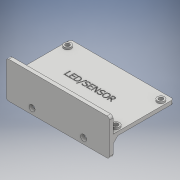
# Autodesk Inventor part: Eletronica - suporteLed
Saved by Autodesk Inventor 2017 (Build 210142000, 142)
## iProperties
Created: 2020-10-10
Part Number: Eletronica - suporteLed
Material: Generic
Document SubType Name: Modeling
Designer: ale
Density: 1 g/cm^3
Appearance: Default
Author: ale
Autodesk Inventor part; units mm, degrees
ref_plane "YZ Plane" through (0, 0, 0) normal (1, 0, 0) x (0, 1, 0)
ref_plane "XZ Plane" through (0, 0, 0) normal (0, 1, 0) x (-1, 0, 0)
ref_plane "XY Plane" through (0, 0, 0) normal (0, 0, 1) x (1, 0, 0)
sketch "Sketch1" plane through (0, 0, 0) normal (0, 0, 1) x (1, 0, 0)
  line L0 (-42.5, 25) -> (42.5, 25)
  line L1 (42.5, 25) -> (42.5, -25)
  line L2 (42.5, -25) -> (-42.5, -25)
  line L3 (-42.5, -25) -> (-42.5, 25)
  line L4 (-42.5, 25) -> (42.5, -25) construction
  line L5 (42.5, 25) -> (-42.5, -25) construction
  point P0 (0, 0)
  dimension "d0" = 85
  dimension "d1" = 50
  constraints: 12 end point, 2 midpoint, 2 parallel, 1 horizontal, 1 perpendicular
  measures "d0" distance of L1.end L2.end
  measures "d1" distance of L0.end L1.end
extrude "Extrusion1" add sketch "Sketch1" along normal blind 3
sketch "Sketch2" plane through (0, 0, 3) normal (0, 0, 1) x (1, 0, 0)
  line L0 (-38.5, 18.5) -> (38.5, 18.5)
  line L1 (38.5, 18.5) -> (38.5, -18.5)
  line L2 (38.5, -18.5) -> (-38.5, -18.5)
  line L3 (-38.5, -18.5) -> (-38.5, 18.5)
  line L4 (-38.5, 18.5) -> (38.5, -18.5) construction
  line L5 (38.5, 18.5) -> (-38.5, -18.5) construction
  circle A0 centre (-38.5, 18.5) radius 3
  circle A1 centre (38.5, 18.5) radius 3
  circle A2 centre (38.5, -18.5) radius 3
  circle A3 centre (-38.5, -18.5) radius 3
  point P0 (0, 0)
  dimension "d30" = 5
  dimension "d4" = 77
  dimension "d5" = 37
  dimension "d6" = 6
  dimension "d7" = 6
  dimension "d8" = 6
  dimension "d9" = 6
  constraints: 12 end point, 4 centre point, 4 coincident, 2 midpoint, 2 parallel, 1 horizontal, 1 perpendicular
  measures "d4" distance of L1.end L2.end
  measures "d5" distance of L0.end L1.end
  measures "d6" diameter of A0
  measures "d7" diameter of A1
  measures "d8" diameter of A2
  measures "d9" diameter of A3
extrude "Extrusion2" add sketch "Sketch2" along normal blind 1.5 contours L3 A0 L0 | L0 A0 L3 | A1 L1 L0 | L0 L1 A1 | A3 L2 L3 | L3 L2 A3 | A2 L2 L1 | L1 L2 A2
sketch "Sketch3" plane through (-38.5, 18.5, 4.5) normal (0, 0, 1) x (1, 0, 0)
  circle A0 centre (0, 0) radius 3 projected
  circle A1 centre (77, 0) radius 3 projected
  circle A2 centre (77, -37) radius 3 projected
  circle A3 centre (0, -37) radius 3 projected
  point P0 (38.5, -18.5)
  constraints: 4 coincident
hole "Hole1" at (-38.5, 18.5, 4.5) at (38.5, 18.5, 4.5) at (38.5, -18.5, 4.5) at (-38.5, -18.5, 4.5) direction (0, 0, -1) diameter 3.5 end through all
sketch "Sketch4" plane through (-42.5, -25, 0) normal (0, -1, 0) x (1, 0, 0)
  line L0 (0, 0) -> (0, 3) projected
  line L1 (0, 1.5) -> (85, 1.5)
  line L2 (85, 0) -> (0, 0) projected
  line L3 (0, 16.5) -> (85, 16.5)
  line L4 (85, 16.5) -> (85, -13.5)
  line L5 (85, -13.5) -> (0, -13.5)
  line L6 (0, -13.5) -> (0, 16.5)
  line L7 (0, 16.5) -> (85, -13.5) construction
  line L8 (85, 16.5) -> (0, -13.5) construction
  point P0 (42.5, 0)
  point P1 (42.5, 1.5)
  dimension "d19" = 85
  dimension "d20" = 30
  constraints: 14 end point, 4 midpoint, 3 parallel, 1 horizontal, 1 perpendicular
  measures "d19" distance of L4.end L5.end
  measures "d20" distance of L3.end L4.end
extrude "Extrusion3" add sketch "Sketch4" along normal blind 3
chamfer "Chamfer1" distance 4 angle 45 1 edges at (0, -25, 0)
sketch "Sketch5" plane through (-42.5, -25, 0) normal (0, 1, 0) x (1, 0, 0)
  line L0 (85, 13.5) -> (0, 13.5) projected
  line L1 (85, 4) -> (85, 13.5) projected
  point P0 (42.5, 0)
  point P1 (63.75, 8.75)
  point P2 (21.25, 8.75)
  dimension "d26" = 4.75
  dimension "d27" = 4.75
  dimension "d28" = 21.25
  dimension "d29" = 63.75
  measures "d26" distance from line of L0 point (63.75, 8.75)
  measures "d27" distance from line of L0 point (21.25, 8.75)
  measures "d28" distance from line of L1 point (63.75, 8.75)
  measures "d29" distance from line of point (21.25, 8.75) L1
hole "Hole2" at (21.25, -25, -8.75) at (-21.25, -25, -8.75) direction (0, -1, 0) diameter 5 end through all
fillet "Fillet1" radius 2 6 edges at (42.5, 25, 1.5) (-42.5, 25, 1.5) (-42.5, -26.5, -13.5) (42.5, -26.5, -13.5) (42.5, -26.5, 16.5) (-42.5, -26.5, 16.5)
sketch "Sketch6" plane through (0, 0, 3) normal (0, 0, 1) x (1, 0, 0)
  line L0 (-20.993, 2.6241) -> (18.8165, 2.6241) construction
  line L1 (18.8165, 2.6241) -> (18.8165, -3.6846) construction
  line L2 (18.8165, -3.6846) -> (-20.993, -3.6846) construction
  line L3 (-20.993, -3.6846) -> (-20.993, 2.6241) construction
  line L4 (-17.5895, -2.5987) -> (-20.4866, -2.5987)
  line L5 (-20.4866, -2.5987) -> (-20.4866, 2.4013)
  line L6 (-20.4866, 2.4013) -> (-19.8221, 2.4013)
  line L7 (-19.8221, 2.4013) -> (-19.8221, -2.0072)
  line L8 (-19.8221, -2.0072) -> (-17.5895, -2.0072)
  line L9 (-17.5895, -2.0072) -> (-17.5895, -2.5987)
  line L10 (-17.0668, -2.5987) -> (-17.0668, 2.4013)
  line L11 (-17.0668, 2.4013) -> (-13.9387, 2.4013)
  line L12 (-13.9387, 2.4013) -> (-13.9387, 1.8097)
  line L13 (-13.9387, 1.8097) -> (-16.4023, 1.8097)
  line L14 (-16.4023, 1.8097) -> (-16.4023, 0.4402)
  line L15 (-16.4023, 0.4402) -> (-14.1049, 0.4402)
  line L16 (-14.1049, 0.4402) -> (-14.1049, -0.1514)
  line L17 (-14.1049, -0.1514) -> (-16.4023, -0.1514)
  line L18 (-16.4023, -0.1514) -> (-16.4023, -2.0072)
  line L19 (-16.4023, -2.0072) -> (-13.9387, -2.0072)
  line L20 (-13.9387, -2.0072) -> (-13.9387, -2.5987)
  line L21 (-13.9387, -2.5987) -> (-17.0668, -2.5987)
  spline S0 degree 2 poles (-9.2669, -0.1028) (-9.2669, -0.7875) (-9.8221, -1.8896) (-10.288, -2.1976) knots 0 0 0 1 2 2 2
  spline S1 degree 2 poles (-10.288, -2.1976) (-10.6689, -2.4366) (-11.4509, -2.5987) (-12.0587, -2.5987) knots 0 0 0 1 2 2 2
  line L22 (-12.0587, -2.5987) -> (-13.2094, -2.5987)
  line L23 (-13.2094, -2.5987) -> (-13.2094, 2.4013)
  line L24 (-13.2094, 2.4013) -> (-12.0708, 2.4013)
  spline S2 degree 2 poles (-12.0708, 2.4013) (-11.3658, 2.4013) (-10.5635, 2.1906) (-10.2799, 2.0042) knots 0 0 0 1 2 2 2
  spline S3 degree 2 poles (-10.2799, 2.0042) (-9.7977, 1.6841) (-9.2669, 0.6266) (-9.2669, -0.1028) knots 0 0 0 1 2 2 2
  spline S4 degree 2 poles (-9.9598, -0.0947) (-9.9598, 0.4807) (-10.3407, 1.2951) (-10.7175, 1.5261) knots 0 0 0 1 2 2 2
  spline S5 degree 2 poles (-10.7175, 1.5261) (-10.9849, 1.6841) (-11.5887, 1.8259) (-12.0384, 1.8259) knots 0 0 0 1 2 2 2
  line L25 (-12.0384, 1.8259) -> (-12.5449, 1.8259)
  line L26 (-12.5449, 1.8259) -> (-12.5449, -2.0234)
  line L27 (-12.5449, -2.0234) -> (-12.0384, -2.0234)
  spline S6 degree 2 poles (-12.0384, -2.0234) (-11.5968, -2.0234) (-10.9282, -1.8815) (-10.6567, -1.6911) knots 0 0 0 1 2 2 2
  spline S7 degree 2 poles (-10.6567, -1.6911) (-10.3083, -1.4561) (-9.9598, -0.6781) (-9.9598, -0.0947) knots 0 0 0 1 2 2 2
  line L28 (-6.6089, 2.6241) -> (-8.566, -3.6846)
  line L29 (-8.566, -3.6846) -> (-9.1332, -3.6846)
  line L30 (-9.1332, -3.6846) -> (-7.1843, 2.6241)
  line L31 (-7.1843, 2.6241) -> (-6.6089, 2.6241)
  spline S8 degree 2 poles (-4.5222, -2.6879) (-5.0652, -2.6879) (-5.8269, -2.461) (-6.1632, -2.2989) knots 0 0 0 1 2 2 2
  line L32 (-6.1632, -2.2989) -> (-6.1632, -1.4642)
  line L33 (-6.1632, -1.4642) -> (-6.1146, -1.4642)
  spline S9 degree 2 poles (-6.1146, -1.4642) (-5.7864, -1.7721) (-4.9558, -2.1125) (-4.5708, -2.1125) knots 0 0 0 1 2 2 2
  spline S10 degree 2 poles (-4.5708, -2.1125) (-4.0198, -2.1125) (-3.4566, -1.6546) (-3.4566, -1.2778) knots 0 0 0 1 2 2 2
  spline S11 degree 2 poles (-3.4566, -1.2778) (-3.4566, -0.978) (-3.7524, -0.6052) (-4.0725, -0.512) knots 0 0 0 1 2 2 2
  spline S12 degree 2 poles (-4.0725, -0.512) (-4.3034, -0.4472) (-4.6883, -0.358) (-4.976, -0.2851) knots 0 0 0 1 2 2 2
  spline S13 degree 2 poles (-4.976, -0.2851) (-5.2353, -0.2162) (-5.6446, -0.0096) (-5.8026, 0.1565) knots 0 0 0 1 2 2 2
  spline S14 degree 2 poles (-5.8026, 0.1565) (-5.9566, 0.3227) (-6.1268, 0.7684) (-6.1268, 1.0601) knots 0 0 0 1 2 2 2
  spline S15 degree 2 poles (-6.1268, 1.0601) (-6.1268, 1.6679) (-5.1786, 2.4904) (-4.4452, 2.4904) knots 0 0 0 1 2 2 2
  spline S16 degree 2 poles (-4.4452, 2.4904) (-4.0238, 2.4904) (-3.2783, 2.3243) (-2.9582, 2.1663) knots 0 0 0 1 2 2 2
  line L34 (-2.9582, 2.1663) -> (-2.9582, 1.3721)
  line L35 (-2.9582, 1.3721) -> (-3.0068, 1.3721)
  spline S17 degree 2 poles (-3.0068, 1.3721) (-3.2459, 1.5909) (-3.9914, 1.9151) (-4.4007, 1.9151) knots 0 0 0 1 2 2 2
  spline S18 degree 2 poles (-4.4007, 1.9151) (-4.8626, 1.9151) (-5.4339, 1.4815) (-5.4339, 1.129) knots 0 0 0 1 2 2 2
  spline S19 degree 2 poles (-5.4339, 1.129) (-5.4339, 0.8129) (-5.0976, 0.4361) (-4.7815, 0.351) knots 0 0 0 1 2 2 2
  spline S20 degree 2 poles (-4.7815, 0.351) (-4.5708, 0.2943) (-3.959, 0.1484) (-3.7564, 0.0877) knots 0 0 0 1 2 2 2
  spline S21 degree 2 poles (-3.7564, 0.0877) (-3.2418, -0.0704) (-2.7637, -0.7065) (-2.7637, -1.1725) knots 0 0 0 1 2 2 2
  spline S22 degree 2 poles (-2.7637, -1.1725) (-2.7637, -1.4683) (-3.0028, -2.0355) (-3.2175, -2.2341) knots 0 0 0 1 2 2 2
  spline S23 degree 2 poles (-3.2175, -2.2341) (-3.4566, -2.4529) (-4.0644, -2.6879) (-4.5222, -2.6879) knots 0 0 0 1 2 2 2
  line L36 (-2.087, -2.5987) -> (-2.087, 2.4013)
  line L37 (-2.087, 2.4013) -> (1.041, 2.4013)
  line L38 (1.041, 2.4013) -> (1.041, 1.8097)
  line L39 (1.041, 1.8097) -> (-1.4225, 1.8097)
  line L40 (-1.4225, 1.8097) -> (-1.4225, 0.4402)
  line L41 (-1.4225, 0.4402) -> (0.8749, 0.4402)
  line L42 (0.8749, 0.4402) -> (0.8749, -0.1514)
  line L43 (0.8749, -0.1514) -> (-1.4225, -0.1514)
  line L44 (-1.4225, -0.1514) -> (-1.4225, -2.0072)
  line L45 (-1.4225, -2.0072) -> (1.041, -2.0072)
  line L46 (1.041, -2.0072) -> (1.041, -2.5987)
  line L47 (1.041, -2.5987) -> (-2.087, -2.5987)
  line L48 (5.3481, -2.5987) -> (4.6026, -2.5987)
  line L49 (4.6026, -2.5987) -> (2.3903, 1.7125)
  line L50 (2.3903, 1.7125) -> (2.3903, -2.5987)
  line L51 (2.3903, -2.5987) -> (1.7703, -2.5987)
  line L52 (1.7703, -2.5987) -> (1.7703, 2.4013)
  line L53 (1.7703, 2.4013) -> (2.7144, 2.4013)
  line L54 (2.7144, 2.4013) -> (4.7282, -1.5574)
  line L55 (4.7282, -1.5574) -> (4.7282, 2.4013)
  line L56 (4.7282, 2.4013) -> (5.3481, 2.4013)
  line L57 (5.3481, 2.4013) -> (5.3481, -2.5987)
  spline S24 degree 2 poles (7.7549, -2.6879) (7.212, -2.6879) (6.4502, -2.461) (6.1139, -2.2989) knots 0 0 0 1 2 2 2
  line L58 (6.1139, -2.2989) -> (6.1139, -1.4642)
  line L59 (6.1139, -1.4642) -> (6.1626, -1.4642)
  spline S25 degree 2 poles (6.1626, -1.4642) (6.4908, -1.7721) (7.3214, -2.1125) (7.7063, -2.1125) knots 0 0 0 1 2 2 2
  spline S26 degree 2 poles (7.7063, -2.1125) (8.2574, -2.1125) (8.8206, -1.6546) (8.8206, -1.2778) knots 0 0 0 1 2 2 2
  spline S27 degree 2 poles (8.8206, -1.2778) (8.8206, -0.978) (8.5248, -0.6052) (8.2047, -0.512) knots 0 0 0 1 2 2 2
  spline S28 degree 2 poles (8.2047, -0.512) (7.9737, -0.4472) (7.5888, -0.358) (7.3011, -0.2851) knots 0 0 0 1 2 2 2
  spline S29 degree 2 poles (7.3011, -0.2851) (7.0418, -0.2162) (6.6326, -0.0096) (6.4745, 0.1565) knots 0 0 0 1 2 2 2
  spline S30 degree 2 poles (6.4745, 0.1565) (6.3206, 0.3227) (6.1504, 0.7684) (6.1504, 1.0601) knots 0 0 0 1 2 2 2
  spline S31 degree 2 poles (6.1504, 1.0601) (6.1504, 1.6679) (7.0985, 2.4904) (7.8319, 2.4904) knots 0 0 0 1 2 2 2
  spline S32 degree 2 poles (7.8319, 2.4904) (8.2533, 2.4904) (8.9989, 2.3243) (9.319, 2.1663) knots 0 0 0 1 2 2 2
  line L60 (9.319, 2.1663) -> (9.319, 1.3721)
  line L61 (9.319, 1.3721) -> (9.2703, 1.3721)
  spline S33 degree 2 poles (9.2703, 1.3721) (9.0313, 1.5909) (8.2857, 1.9151) (7.8765, 1.9151) knots 0 0 0 1 2 2 2
  spline S34 degree 2 poles (7.8765, 1.9151) (7.4146, 1.9151) (6.8433, 1.4815) (6.8433, 1.129) knots 0 0 0 1 2 2 2
  spline S35 degree 2 poles (6.8433, 1.129) (6.8433, 0.8129) (7.1796, 0.4361) (7.4956, 0.351) knots 0 0 0 1 2 2 2
  spline S36 degree 2 poles (7.4956, 0.351) (7.7063, 0.2943) (8.3181, 0.1484) (8.5207, 0.0877) knots 0 0 0 1 2 2 2
  spline S37 degree 2 poles (8.5207, 0.0877) (9.0353, -0.0704) (9.5134, -0.7065) (9.5134, -1.1725) knots 0 0 0 1 2 2 2
  spline S38 degree 2 poles (9.5134, -1.1725) (9.5134, -1.4683) (9.2744, -2.0355) (9.0596, -2.2341) knots 0 0 0 1 2 2 2
  spline S39 degree 2 poles (9.0596, -2.2341) (8.8206, -2.4529) (8.2128, -2.6879) (7.7549, -2.6879) knots 0 0 0 1 2 2 2
  spline S40 degree 2 poles (13.7274, 1.83) (14.011, 1.4977) (14.3271, 0.5253) (14.3271, -0.0987) knots 0 0 0 1 2 2 2
  spline S41 degree 2 poles (14.3271, -0.0987) (14.3271, -0.7065) (14.0191, -1.6911) (13.7274, -2.0234) knots 0 0 0 1 2 2 2
  spline S42 degree 2 poles (13.7274, -2.0234) (13.4194, -2.3718) (12.605, -2.7041) (12.1147, -2.7041) knots 0 0 0 1 2 2 2
  spline S43 degree 2 poles (12.1147, -2.7041) (11.6083, -2.7041) (10.7979, -2.3597) (10.5021, -2.0234) knots 0 0 0 1 2 2 2
  spline S44 degree 2 poles (10.5021, -2.0234) (10.2144, -1.6911) (9.9065, -0.7146) (9.9065, -0.0987) knots 0 0 0 1 2 2 2
  spline S45 degree 2 poles (9.9065, -0.0987) (9.9065, 0.5293) (10.2185, 1.4856) (10.5061, 1.83) knots 0 0 0 1 2 2 2
  spline S46 degree 2 poles (10.5061, 1.83) (10.7979, 2.1622) (11.6123, 2.5066) (12.1147, 2.5066) knots 0 0 0 1 2 2 2
  spline S47 degree 2 poles (12.1147, 2.5066) (12.6253, 2.5066) (13.4438, 2.1501) (13.7274, 1.83) knots 0 0 0 1 2 2 2
  spline S48 degree 2 poles (13.6342, -0.0987) (13.6342, 0.3956) (13.4194, 1.1614) (13.225, 1.4126) knots 0 0 0 1 2 2 2
  spline S49 degree 2 poles (13.225, 1.4126) (13.0264, 1.6719) (12.4673, 1.9313) (12.1188, 1.9313) knots 0 0 0 1 2 2 2
  spline S50 degree 2 poles (12.1188, 1.9313) (11.7582, 1.9313) (11.2152, 1.68) (11.0086, 1.4126) knots 0 0 0 1 2 2 2
  spline S51 degree 2 poles (11.0086, 1.4126) (10.81, 1.1574) (10.5993, 0.3875) (10.5993, -0.0987) knots 0 0 0 1 2 2 2
  spline S52 degree 2 poles (10.5993, -0.0987) (10.5993, -1.0833) (11.4259, -2.1287) (12.1188, -2.1287) knots 0 0 0 1 2 2 2
  spline S53 degree 2 poles (12.1188, -2.1287) (12.8117, -2.1287) (13.6342, -1.0833) (13.6342, -0.0987) knots 0 0 0 1 2 2 2
  line L62 (18.9259, -2.5987) -> (18.0629, -2.5987)
  line L63 (18.0629, -2.5987) -> (16.4826, -0.6093)
  line L64 (16.4826, -0.6093) -> (15.7209, -0.6093)
  line L65 (15.7209, -0.6093) -> (15.7209, -2.5987)
  line L66 (15.7209, -2.5987) -> (15.0564, -2.5987)
  line L67 (15.0564, -2.5987) -> (15.0564, 2.4013)
  line L68 (15.0564, 2.4013) -> (16.3449, 2.4013)
  spline S54 degree 2 poles (16.3449, 2.4013) (16.7744, 2.4013) (17.3538, 2.3081) (17.6172, 2.1379) knots 0 0 0 1 2 2 2
  spline S55 degree 2 poles (17.6172, 2.1379) (17.8805, 1.9677) (18.1844, 1.4369) (18.1844, 1.0439) knots 0 0 0 1 2 2 2
  spline S56 degree 2 poles (18.1844, 1.0439) (18.1844, 0.4969) (17.6253, -0.2446) (17.1472, -0.4229) knots 0 0 0 1 2 2 2
  line L69 (17.1472, -0.4229) -> (18.9259, -2.5987)
  spline S57 degree 2 poles (17.4916, 0.9912) (17.4916, 1.21) (17.3376, 1.5463) (17.1755, 1.6557) knots 0 0 0 1 2 2 2
  spline S58 degree 2 poles (17.1755, 1.6557) (17.0337, 1.7489) (16.6569, 1.8259) (16.3814, 1.8259) knots 0 0 0 1 2 2 2
  line L70 (16.3814, 1.8259) -> (15.7209, 1.8259)
  line L71 (15.7209, 1.8259) -> (15.7209, -0.0542)
  line L72 (15.7209, -0.0542) -> (16.3044, -0.0542)
  spline S59 degree 2 poles (16.3044, -0.0542) (16.592, -0.0542) (17.0499, 0.0471) (17.2079, 0.2052) knots 0 0 0 1 2 2 2
  spline S60 degree 2 poles (17.2079, 0.2052) (17.3538, 0.3429) (17.4916, 0.7319) (17.4916, 0.9912) knots 0 0 0 1 2 2 2
  point P0 (0, 0)
  constraints: 2 other
emboss "Emboss1" sketch "Sketch6" operation cut depth 1 direction (0, 0, -1)
body "Solid1"
